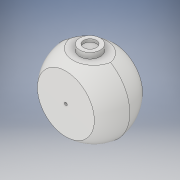
# Autodesk Inventor part: Part1
Saved by Autodesk Inventor 2017 (Build 210142000, 142)
## iProperties
Created: 2020-02-20
Part Number: Part1
Material: UHMW, White
Document SubType Name: Modeling
Designer: S346852600
Density: 0.94 g/cm^3
Appearance: Smooth - White
Author: S346852600
Autodesk Inventor part; units mm, degrees
ref_plane "YZ Plane" through (0, 0, 0) normal (1, 0, 0) x (0, 1, 0)
ref_plane "XZ Plane" through (0, 0, 0) normal (0, 1, 0) x (-1, 0, 0)
ref_plane "XY Plane" through (0, 0, 0) normal (0, 0, 1) x (1, 0, 0)
sketch "Sketch1" plane through (0, 0, 0) normal (1, 0, 0) x (0, 1, 0)
  line L0 (0, 0) -> (0, 43.1038)
  line L1 (0, 21.5519) -> (35.56, 21.5519)
  line L2 (0, 43.1038) -> (25.4, 43.1038)
  line L3 (0, 0) -> (25.4, 0)
  arc A0 (25.4, 0) -> (35.56, 21.5519) centre (0.1738, 25.0629) ccw
  arc A1 (35.56, 21.5519) -> (25.4, 43.1038) centre (0.1738, 18.0409) ccw
  dimension "d0" = 43.1038
  dimension "d1" = 35.56
  dimension "d2" = 25.4
  dimension "d4" = 25.4
  dimension "d5" = 35.56
  dimension "d6" = 35.56
  constraints: 8 end point, 4 point on circle, 3 horizontal, 2 centre point, 1 midpoint, 1 vertical
  measures "d0" distance of L0.start L0.end
  measures "d1" distance of L1.start L1.end
  measures "d2" distance of L0.end L2.end
  measures "d4" distance of L0.start L3.end
  measures "d5" radius of A0
  measures "d6" radius of A1
revolve "Revolution2" add sketch "Sketch1" angle 360 about axis through (0, 0, 0) along (0, 0, 1)
sketch "Sketch3" plane through (0, 0, 0) normal (0, 0, -1) x (-1, 0, 0)
  circle A0 centre (0, 0) radius 25.4 projected
  line L0 (0, 0) -> (0, 30.48)
  line L1 (0, 30.48) -> (9.144, 30.48)
  line L2 (9.144, 30.48) -> (18.3162, 30.48)
  circle A1 centre (0, 0) radius 35.56 projected
  line L3 (0, 30.48) -> (-18.3162, 30.48)
  line L4 (0, 30.48) -> (0, 35.56)
  arc A2 (0, 35.56) -> (-18.3162, 30.48) centre (0, 0) ccw
  arc A3 (18.3162, 30.48) -> (0, 35.56) centre (0, 0) ccw
  dimension "d11" = 30.48
  dimension "d12" = 9.144
  constraints: 10 end point, 7 point on circle, 3 concentric, 2 centre point, 2 perpendicular, 1 horizontal, 1 point on line, 1 vertical
  measures "d11" distance of L0.start L0.end
  measures "d12" distance of L0.end L1.end
extrude "Extrusion1" cut sketch "Sketch3" against normal blind 47.625 contours L3 A1 L4 | L4 A1 L2 L1
sketch "Sketch4" plane through (0, 30.48, 29.0975) normal (0, 1, 0) x (0.9819, 0, -0.1892)
  line L0 (-16.5583, 10.874) -> (19.4128, 3.9448)
  line L1 (36.3453, 0.6831) -> (-33.4908, 14.1357) projected
  circle A0 centre (1.4273, 7.4094) radius 9.271
  point P0 (5.5039, 28.5723)
  dimension "d15" = 18.542
  constraints: 2 end point, 1 centre point, 1 collinear, 1 midpoint
  measures "d15" diameter of A0
extrude "Extrusion2" add sketch "Sketch4" along normal blind 5.08
sketch "Sketch5" plane through (0, 35.56, 21.5519) normal (0, 1, 0) x (1, 0, 0)
  line L0 (35.56, 0) -> (-35.56, 0) projected
  circle A0 centre (0, 0) radius 5.715
  point P0 (0, 21.5519)
  point P1 (18.3162, 0)
  point P2 (-18.3162, 0)
  dimension "d18" = 11.43
  constraints: 1 centre point, 1 midpoint
  measures "d18" diameter of A0
extrude "Extrusion3" cut sketch "Sketch5" against normal blind 2.54
sketch "Sketch6" plane through (0, 0, 0) normal (0, 0, -1) x (-1, 0, 0)
  circle A0 centre (0, 0) radius 1.27
  dimension "d21" = 2.54
  constraints: 1 centre point, 1 coincident
  measures "d21" diameter of A0
sketch "Sketch7" plane through (0, 0, 43.1038) normal (0, 0, 1) x (1, 0, 0)
  circle A0 centre (0, 0) radius 1.27
  dimension "d22" = 2.54
  constraints: 1 centre point, 1 coincident
  measures "d22" diameter of A0
extrude "Extrusion4" cut sketch "Sketch6" against normal blind 2.54
extrude "Extrusion5" cut sketch "Sketch7" against normal blind 2.54
body "Solid2"
